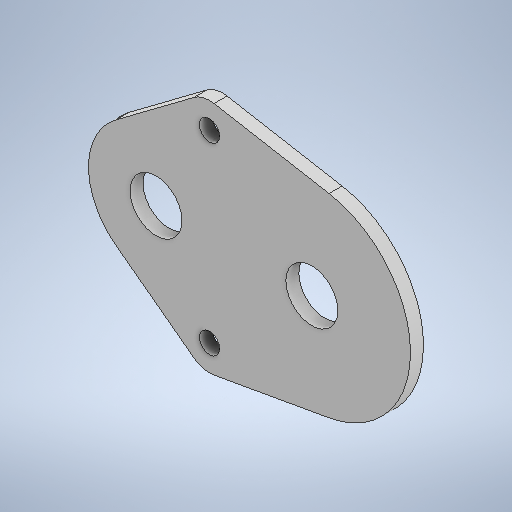
# Autodesk Inventor part: Gearbox plate #1
Saved by Autodesk Inventor 2025.1 (Build 291241020, 241B)
## iProperties
Created: 2024-09-08
Part Number: Gearbox plate #1
Material: Generic
Document SubType Name: Modeling
Designer: xmand
Density: 1 g/cm^3
Appearance: Default
Author: xmand
Autodesk Inventor part; units mm, degrees
ref_plane "YZ Plane" through (0, 0, 0) normal (1, 0, 0) x (0, 1, 0)
ref_plane "XZ Plane" through (0, 0, 0) normal (0, 1, 0) x (-1, 0, 0)
ref_plane "XY Plane" through (0, 0, 0) normal (0, 0, 1) x (1, 0, 0)
sketch "Sketch1" plane through (0, 0, 0) normal (0, 0, 1) x (1, 0, 0)
  circle A0 centre (0, 0) radius 22.86 construction
  circle A1 centre (-38.1, 0) radius 15.24 construction
  circle A2 centre (0, 0) radius 24.13 construction
  circle A3 centre (-38.1, 0) radius 16.51 construction
  circle A4 centre (-25.019, -22.5102) radius 6.35 construction
  line L0 (-29.8047, -14.2748) -> (-28.2095, -17.0199) construction
  line L1 (-17.9382, -16.1394) -> (-20.2984, -18.263) construction
  circle A5 centre (-38.1, 0) radius 6.35
  circle A6 centre (0, 0) radius 6.35
  line L2 (-28.8289, -27.5903) -> (-48.0058, -13.2082)
  line L3 (-23.9068, -28.762) -> (4.2265, -23.757)
  arc A7 (-48.0058, 13.2082) -> (-48.0058, -13.2082) centre (-38.1, 0) ccw
  arc A8 (4.2265, -23.757) -> (4.2265, 23.757) centre (0, 0) ccw
  arc A9 (-28.8289, -27.5903) -> (-23.9068, -28.762) centre (-25.019, -22.5102) ccw
  circle A10 centre (-25.019, -22.5102) radius 2.4892
  circle A11 centre (-25.019, 22.5102) radius 6.35 construction
  line L4 (-17.9382, 16.1394) -> (-20.2984, 18.263) construction
  line L5 (-28.2095, 17.0199) -> (-29.8047, 14.2748) construction
  line L6 (4.2265, 23.757) -> (-23.9068, 28.762)
  line L7 (-28.8289, 27.5903) -> (-48.0058, 13.2082)
  arc A12 (-23.9068, 28.762) -> (-28.8289, 27.5903) centre (-25.019, 22.5102) ccw
  circle A13 centre (-25.019, 22.5102) radius 2.4892
  dimension "d3" = 30.48
  dimension "d4" = 45.72
  dimension "d5" = 48.26
  dimension "d6" = 33.02
  dimension "d23" = 12.7
  dimension "d30" = 12.7
  dimension "d31" = 12.7
  dimension "d33" = 3.175
  dimension "d34" = 3.175
  dimension "d35" = 4.9784
  dimension "d36" = 12.7
  dimension "d37" = 3.175
  dimension "d38" = 3.175
  dimension "d39" = 4.9784
  constraints: 24 point on circle, 16 end point, 14 centre point, 12 tangent, 8 coincident, 8 point on line, 2 concentric, 2 horizontal alignment
  measures "d3" diameter of A1
  measures "d4" diameter of A0
  measures "d5" diameter of A2
  measures "d6" diameter of A3
  measures "d23" diameter of A4
  measures "d30" diameter of A5
  measures "d31" diameter of A6
  measures "d33" distance of L1.end L1.start
  measures "d34" distance of L0.start L0.end
  measures "d35" diameter of A10
  measures "d36" diameter of A11
  measures "d37" distance of L4.start L4.end
  measures "d38" distance of L5.start L5.end
  measures "d39" diameter of A13
extrude "Extrusion1" add sketch "Sketch1" along normal mid plane 3.175
body "Solid1"
